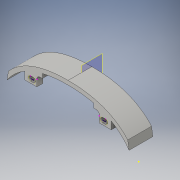
# Autodesk Inventor part: bumper
Saved by Autodesk Inventor 2016 (Build 200138000, 138)
## iProperties
Created: 2015-09-30
Part Number: bumper
Material: Generic
Document SubType Name: Modeling
Designer: Jesse Stevenson
Density: 1 g/cm^3
Appearance: Default
Author: Jesse Stevenson
Autodesk Inventor part; units mm, degrees
ref_plane "YZ Plane" through (0, 0, 0) normal (1, 0, 0) x (0, 1, 0)
ref_plane "XZ Plane" through (0, 0, 0) normal (0, 1, 0) x (-1, 0, 0)
ref_plane "XY Plane" through (0, 0, 0) normal (0, 0, 1) x (1, 0, 0)
ref_plane "Work Plane1" through (-51.8377, -68.0226, 19.9348) normal (1, 0, 0) x (0, -1, 0)
sketch "Sketch4" plane through (0, 0, 0) normal (0, 0, 1) x (1, 0, 0)
  line L0 (-75.4685, 56.7135) -> (-75.4685, -159.0824) construction
  line L1 (-75.4685, 33.1535) -> (-121.7477, 33.1535) construction
  line L2 (-121.7477, 33.1535) -> (-140.5673, 5.3749) construction
  spline S0 degree 2 poles (-75.4685, 33.1535) (-121.7477, 33.1535) (-140.5673, 5.3749) knots 1 1 1 2 2 2
  line L3 (-75.4685, 33.1535) -> (-29.1892, 33.1535) construction
  line L4 (-29.1892, 33.1535) -> (-10.3697, 5.3749) construction
  spline S1 degree 2 poles (-75.4685, 33.1535) (-29.1892, 33.1535) (-10.3697, 5.3749) knots 1 1 1 2 2 2
  line L5 (-11.812, 14.2406) -> (-10.3697, 5.3749)
  line L6 (-140.5673, 5.3749) -> (-139.125, 14.2406)
  spline S2 degree 5 poles (-11.8119, 14.2406) (-13.8893, 16.5679) (-16.1177, 18.7603) (-18.4876, 20.803) (-25.009, 25.725) (-32.2587, 29.5483) (-36.9345, 31.4831) (-47.2853, 34.8351) (-58.027, 36.6239) (-63.8293, 37.2041) (-69.6491, 37.4715) (-75.4685, 37.4715) knots 0 0 0 0 0 0 0.223232 0.223232 0.223232 0.583566 0.583566 0.583566 1 1 1 1 1 1
  spline S3 degree 5 poles (-75.4685, 37.4715) (-81.2878, 37.4715) (-87.1077, 37.2041) (-92.91, 36.6239) (-103.6516, 34.8351) (-114.0025, 31.4831) (-118.6782, 29.5483) (-125.9279, 25.725) (-132.4493, 20.803) (-134.8192, 18.7603) (-137.0476, 16.5679) (-139.125, 14.2406) knots 0 0 0 0 0 0 0.416434 0.416434 0.416434 0.776768 0.776768 0.776768 1 1 1 1 1 1
  point P0 (0, 0)
  dimension "d7" = 4.318
  constraints: 6 end point, 2 symmetric about line, 1 perpendicular, 1 point on line, 1 vertical, 14 other
extrude "Extrusion3" add sketch "Sketch4" along normal blind 25.4
sketch "Sketch5" plane through (0, 0, 25.4) normal (0, 0, 1) x (1, 0, 0)
  circle A0 centre (-38.6912, 19.3223) radius 1.7859
  spline S0 degree 2 poles (-140.5673, 5.3749) (-121.7477, 33.1535) (-75.4685, 33.1535) knots 0 0 0 1 1 1 projected
  spline S1 degree 2 poles (-75.4685, 33.1535) (-29.1892, 33.1535) (-10.3697, 5.3749) knots 0 0 0 1 1 1 projected
  line L0 (-10.3697, 5.3749) -> (-11.812, 14.2406) construction
  line L1 (-139.125, 14.2406) -> (-140.5673, 5.3749) construction
  line L2 (-75.4685, 33.1535) -> (-75.4685, 27.4661) construction
  line L3 (-18.3678, 14.7921) -> (-47.9923, 14.7921)
  line L4 (-47.9923, 14.7921) -> (-47.9923, 30.1475)
  line L5 (-38.6912, 19.3223) -> (-35.3861, 19.3223) construction
  line L6 (-38.6912, 21.7659) -> (-35.3861, 21.7659)
  line L7 (-35.3861, 16.8787) -> (-38.6912, 16.8787)
  arc A1 (-38.6912, 21.7659) -> (-38.6912, 16.8787) centre (-38.6912, 19.3223) ccw
  arc A2 (-35.3861, 16.8787) -> (-35.3861, 21.7659) centre (-35.3861, 19.3223) ccw
  circle A3 centre (-112.2458, 19.3223) radius 1.7859
  line L8 (-102.9446, 14.7921) -> (-102.9446, 30.1475)
  line L9 (-112.2458, 19.3223) -> (-115.5508, 19.3223) construction
  line L10 (-112.2458, 21.7659) -> (-115.5508, 21.7659)
  line L11 (-115.5508, 16.8787) -> (-112.2458, 16.8787)
  arc A4 (-112.2458, 16.8787) -> (-112.2458, 21.7659) centre (-112.2458, 19.3223) ccw
  arc A5 (-115.5508, 21.7659) -> (-115.5508, 16.8787) centre (-115.5508, 19.3223) ccw
  line L12 (-102.9446, 14.7921) -> (-132.5692, 14.7921)
  circle A6 centre (-35.3861, 19.3223) radius 1.7859 construction
  point P0 (0, 0)
  point P1 (-37.0387, 19.3223)
  point P2 (-113.8983, 19.3223)
  constraints: 26 end point, 9 symmetric about line, 8 point on circle, 6 centre point, 4 tangent, 3 horizontal, 2 vertical, 1 coincident, 1 equal radius, 1 midpoint, 1 parallel, 11 other
extrude "Extrusion4" add sketch "Sketch5" against normal blind 6.35 contours S0 L8 L12 | S1 L3 L4
sketch "Sketch6" plane through (0, 0, 25.4) normal (0, 0, 1) x (1, 0, 0)
  arc A0 (-38.6912, 21.7659) -> (-38.6912, 16.8787) centre (-38.6912, 19.3223) ccw construction
  arc A1 (-35.3861, 16.8787) -> (-35.3861, 21.7659) centre (-35.3861, 19.3223) ccw construction
  line L0 (-38.6912, 19.3223) -> (-35.3861, 19.3223)
  point P0 (0, 0)
  point P1 (-42.1313, 21.6591)
  point P2 (-35.4929, 21.6591)
  constraints: 2 end point, 1 horizontal, 2 other
sketch "Sketch7" plane through (0, 0, 25.4) normal (0, 0, 1) x (1, 0, 0)
  arc A0 (-115.5508, 21.7659) -> (-115.5508, 16.8787) centre (-115.5508, 19.3223) ccw construction
  arc A1 (-112.2458, 16.8787) -> (-112.2458, 21.7659) centre (-112.2458, 19.3223) ccw construction
  line L0 (-115.5508, 19.3223) -> (-112.2458, 19.3223)
  point P0 (0, 0)
  point P1 (-115.444, 21.6591)
  point P2 (-108.8057, 21.6591)
  constraints: 2 end point, 1 horizontal, 2 other
sketch "Sketch8" plane through (0, 0, 19.05) normal (0, 0, -1) x (-1, 0, 0)
  spline S0 degree 2 poles (75.4685, 33.1535) (121.7477, 33.1535) (140.5673, 5.3749) knots 0 0 0 1 1 1 projected
  line L0 (102.9446, 14.7921) -> (132.5692, 14.7921) projected
  line L1 (121.5357, 14.7921) -> (121.5357, 22.9175)
  point P0 (0, 0)
  constraints: 2 end point, 1 point on line, 1 vertical, 2 other
extrude "Extrusion5" cut sketch "Sketch8" against normal through all
ref_plane "Work Plane3" through (-75.4685, 33.1535, 0) normal (-1, 0, 0) x (0, -1, 0)
mirror "Mirror1" about plane through (-75.4685, 33.1535, 0) normal (-1, 0, 0) of "Extrusion5"
sketch "Sketch9" plane through (0, 0, 25.4) normal (0, 0, 1) x (1, 0, 0)
  line L0 (-47.9923, 14.7921) -> (-29.4013, 14.7921) projected
  line L1 (-47.9923, 14.7921) -> (-42.1245, 14.7921)
  line L2 (-42.1245, 14.7921) -> (-42.1245, 22.3222)
  line L3 (-45.2995, 25.4972) -> (-47.9923, 25.4972)
  line L4 (-47.9923, 25.4972) -> (-47.9923, 14.7921)
  arc A0 (-42.1245, 22.3222) -> (-45.2995, 25.4972) centre (-45.2995, 22.3222) ccw
  point P0 (0, 0)
  dimension "d20" = 3.175
  constraints: 8 end point, 2 parallel, 2 point on circle, 2 tangent, 1 centre point, 1 horizontal, 1 perpendicular
  measures "d20" radius of A0
extrude "Extrusion6" cut sketch "Sketch9" against normal through all
mirror "Mirror2" about plane through (-75.4685, 33.1535, 0) normal (-1, 0, 0) of "Extrusion6"
body "Solid2"
